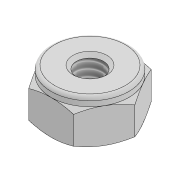
# Autodesk Inventor part: 10_028_NYLON_NUT_M2_R1
Saved by Autodesk Inventor 2021.2 (Build 252289000, 289)
## iProperties
Created: 2021-01-15
Part Number: 10_028_NYLON_NUT_M2_R1
Material: Generic
Document SubType Name: Modeling
Designer: y6tada
Density: 1 g/cm^3
Appearance: Default
Author: y6tada
Autodesk Inventor part; units mm, degrees
ref_plane "YZ Plane" through (0, 0, 0) normal (1, 0, 0) x (0, 1, 0)
ref_plane "XZ Plane" through (0, 0, 0) normal (0, 1, 0) x (-1, 0, 0)
ref_plane "XY Plane" through (0, 0, 0) normal (0, 0, 1) x (1, 0, 0)
sketch "Sketch1" plane through (0, 0, 0) normal (0, 1, 0) x (-1, 0, 0)
  line L0 (-2.5981, 0) -> (-1.299, 2.25)
  line L1 (-1.299, 2.25) -> (1.299, 2.25)
  line L2 (1.299, 2.25) -> (2.5981, 0)
  line L3 (2.5981, 0) -> (1.299, -2.25)
  line L4 (1.299, -2.25) -> (-1.299, -2.25)
  line L5 (-1.299, -2.25) -> (-2.5981, 0)
  point P0 (0, 0)
  point P1 (0, 0)
  dimension "d0" = 4.5
  constraints: 12 end point, 1 coincident, 1 horizontal, 13 other
  measures "d0" distance between parallel lines of L1 L4
extrude "Extrusion1" add sketch "Sketch1" along normal blind 2.5
sketch "Sketch2" plane through (0, 0, 0) normal (1, 0, 0) x (0, 1, 0)
  line L0 (0, -2.25) -> (0, 0) construction
  line L1 (2.5, -2.25) -> (2.5, 0) construction
  line L2 (0, -2.25) -> (0, -5.0728)
  line L3 (0, -5.0728) -> (1.6297, -5.0728)
  line L4 (1.6297, -5.0728) -> (0, -2.25)
  line L5 (2.5, -2.25) -> (2, -2.25)
  line L6 (2, -2.25) -> (1.5484, -3.0322)
  line L7 (1.5484, -3.0322) -> (2.5, -3.0322)
  line L8 (2.5, -3.0322) -> (2.5, -2.25)
  line L9 (0, -2.25) -> (2.5, -2.25) construction
  line L10 (0, 0) -> (3.5883, 0) construction
  dimension "d4" = 30
  dimension "d5" = 2
  dimension "d6" = 30
  dimension "d7" = 4.5
  constraints: 16 end point, 3 point on line, 2 horizontal, 2 vertical, 1 parallel, 1 perpendicular
  measures "d4" angle of L2 L4
  measures "d5" distance of L0.start point (2, -2.25)
  measures "d6" angle of L6 L8
  measures "d7" diameter of L5 L10
revolve "Revolution1" cut sketch "Sketch2" angle 360 about axis through (0, 0, 0) along (0, 1, 0)
fillet "Fillet1" radius 0.2 1 edges at (0, 2.5, 2.25)
sketch "Sketch4" plane through (0, 0, 0) normal (0, -1, 0) x (1, 0, 0)
  point P0 (0, 0)
  point P1 (0, 0)
  constraints: 1 coincident
hole "Hole1" at (0, 0, 0) direction (0, 1, 0) diameter 1.567 end through all thread size "M2x0.4" class "6H" standard "ANSI Metric M Profile"
chamfer "Chamfer1" distance 0.2 angle 45 2 edges at (0, 2.5, 0.7835) (0, 0, 0.7835)
body "Solid1"
